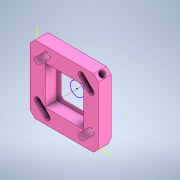
# Autodesk Inventor part: 20_Cube_Insert_Kinematic_Beautymirrormount_90_pro_v3
Saved by Autodesk Inventor 2022 (Build 260153000, 153)
## iProperties
Created: 2021-11-15
Part Number: 20_Cube_Insert_Kinematic_Beautymirrormount_90_pro_v3
Material: Generic
Document SubType Name: Modeling
Designer: diederichbenedict
Density: 1 g/cm^3
Appearance: Pink
Author: diederichbenedict
Autodesk Inventor part; units mm, degrees
ref_plane "YZ Plane" through (0, 0, 0) normal (1, 0, 0) x (0, 1, 0)
ref_plane "XY Plane" through (0, 0, 0) normal (0, 0, 1) x (1, 0, 0)
ref_plane "Work Plane1" through (0, 0, 2) normal (0, 0, 1) x (1, 0, 0)
sketch "Sketch1" plane through (0, 0, 2) normal (0, 0, 1) x (1, 0, 0)
  circle A0 centre (-37.0712, 14) radius 3.25 construction
  circle A1 centre (-9.0712, -14) radius 3.25 construction
  line L0 (-26.0712, -17.08) -> (-20.0712, -17.08) construction
  arc A2 (-20.0712, -17.08) -> (-20.0712, -14.08) centre (-20.0712, -15.58) ccw construction
  line L1 (-20.0712, -14.08) -> (-26.0712, -14.08) construction
  line L2 (-37.0712, -3) -> (-37.0712, 3) construction
  arc A3 (-37.0712, 3) -> (-40.0712, 3) centre (-38.5712, 3) ccw construction
  line L3 (-40.0712, 3) -> (-40.0712, -3) construction
  line L4 (-47.9712, -17) -> (-47.9712, 17) construction
  line L5 (-47.9712, 17) -> (-44.3964, 17) construction
  line L6 (-44.3964, 17) -> (-40.0712, 21.3252) construction
  line L7 (-40.0712, 21.3252) -> (-40.0712, 24.9) construction
  line L8 (-40.0712, 24.9) -> (-6.0712, 24.9) construction
  line L9 (-6.0712, 24.9) -> (-6.0712, 21.3252) construction
  line L10 (-6.0712, 21.3252) -> (-1.746, 17) construction
  line L11 (-1.746, 17) -> (1.8288, 17) construction
  line L12 (1.8288, 17) -> (1.8288, -17) construction
  line L13 (1.8288, -17) -> (-1.746, -17) construction
  line L14 (-1.746, -17) -> (-6.1126, -21.3666) construction
  line L15 (-6.1126, -21.3666) -> (-6.1126, -24.9) construction
  line L16 (-6.1126, -24.9) -> (-40.0712, -24.9) construction
  circle A4 centre (-37.0712, -14) radius 3.25 construction
  circle A5 centre (-23.0712, 0) radius 12.45 construction
  circle A6 centre (-23.0712, 0) radius 12.7 construction
  line L17 (-37.0712, 14) -> (-9.0712, 14) construction
  line L18 (-9.0712, 14) -> (-9.0712, -14) construction
  line L19 (-9.0712, -14) -> (-37.0712, -14) construction
  line L20 (-37.0712, -14) -> (-37.0712, 14) construction
  line L21 (-4.0712, -19) -> (-4.0712, 19)
  line L22 (-4.0712, 19) -> (-42.0712, 19)
  line L23 (-42.0712, 19) -> (-42.0712, -19)
  line L24 (-42.0712, -19) -> (-4.0712, -19)
  circle A7 centre (-23.0712, 0) radius 12.8
  circle A8 centre (-23.0712, 0) radius 3.25 projected
  line L25 (-40.0712, -24.9) -> (-40.0712, -21.3252) projected
  line L26 (-40.0712, -21.3252) -> (-44.3964, -17) projected
  line L27 (-44.3964, -17) -> (-47.9712, -17) projected
  arc A9 (-26.0712, -14.08) -> (-26.0712, -17.08) centre (-26.0712, -15.58) ccw projected
  arc A10 (-40.0712, -3) -> (-37.0712, -3) centre (-38.5712, -3) ccw projected
  circle A11 centre (-37.0712, -14) radius 3.25 projected
  point P0 (0, 0)
  point P1 (-21.8762, -3.0223)
  point P2 (-25.9925, 1.4242)
  dimension "d0" = 5
  dimension "d1" = 0.1
  constraints: 16 end point, 4 parallel, 2 perpendicular, 1 centre point, 1 horizontal, 3 other
  measures "d0" distance between parallel lines of L18 L21
  measures "d1" radial gap between concentric circles of A6 A7
extrude "Extrusion1" add sketch "Sketch1" along normal blind 6 contours L24 L23 L22 L21 | A7 | A11
sketch "Sketch2" plane through (0, 0, 2) normal (0, 0, -1) x (-1, 0, 0)
  circle A0 centre (23.0712, 0) radius 12.8 projected
  circle A1 centre (23.0712, 0) radius 8.5824
  point P0 (0, 0)
  constraints: 1 centre point
extrude "Extrusion2" add sketch "Sketch2" against normal blind 0.5
sketch "Sketch3" plane through (0, 0, 2) normal (0, 0, -1) x (-1, 0, 0)
  circle A0 centre (9.0712, -14) radius 1.45 construction
  circle A1 centre (9.0712, -14) radius 2.45
  circle A2 centre (37.0712, -14) radius 1.45 projected
  circle A3 centre (37.0712, -14) radius 1.95
  point P0 (0, 0)
  dimension "d8" = 1
  dimension "d10" = 0.5
  constraints: 2 centre point
  measures "d8" radial gap between concentric circles of A0 A1
  measures "d10" radial gap between concentric circles of A2 A3
sketch "Sketch5" plane through (0, 0, 2) normal (0, 0, -1) x (-1, 0, 0)
  arc A0 (20.0712, -14.08) -> (20.0712, -17.08) centre (20.0712, -15.58) ccw construction
  arc A1 (26.0712, -17.08) -> (26.0712, -14.08) centre (26.0712, -15.58) ccw construction
  line L0 (37.0712, 3) -> (37.0712, -3) projected
  arc A2 (37.0712, -3) -> (40.0712, -3) centre (38.5712, -3) ccw projected
  line L1 (40.0712, -3) -> (40.0712, 3) projected
  arc A3 (40.0712, 3) -> (37.0712, 3) centre (38.5712, 3) ccw projected
  line L2 (26.0712, -14.08) -> (20.0712, -14.08) construction
  arc A4 (20.0712, -14.08) -> (20.0712, -17.08) centre (20.0712, -15.58) ccw construction
  line L3 (20.0712, -17.08) -> (26.0712, -17.08) construction
  arc A5 (26.0712, -17.08) -> (26.0712, -14.08) centre (26.0712, -15.58) ccw construction
  circle A6 centre (37.0712, -14) radius 1.45 projected
  circle A7 centre (23.0712, 0) radius 1.45 projected
  circle A8 centre (9.0712, -14) radius 1.45 projected
  circle A9 centre (37.0712, 14) radius 1.45 projected
  line L4 (-1.8288, -17) -> (-1.8288, 17) projected
  line L5 (-1.8288, 17) -> (1.746, 17) projected
  line L6 (1.746, 17) -> (6.0712, 21.3252) projected
  line L7 (6.0712, 21.3252) -> (6.0712, 24.9) projected
  line L8 (6.0712, 24.9) -> (40.0712, 24.9) projected
  line L9 (40.0712, 24.9) -> (40.0712, 21.3252) projected
  line L10 (40.0712, 21.3252) -> (44.3964, 17) projected
  line L11 (44.3964, 17) -> (47.9712, 17) projected
  line L12 (47.9712, 17) -> (47.9712, -17) projected
  line L13 (44.3964, -17) -> (47.9712, -17) projected
  line L14 (40.0712, -21.3252) -> (44.3964, -17) projected
  line L15 (40.0712, -24.9) -> (40.0712, -21.3252) projected
  line L16 (6.1126, -24.9) -> (40.0712, -24.9) projected
  line L17 (6.1126, -24.9) -> (6.1126, -21.3666) projected
  line L18 (6.1126, -21.3666) -> (1.746, -17) projected
  line L19 (1.746, -17) -> (-1.8288, -17) projected
  line L20 (42.0712, -19) -> (4.0712, -19) projected
  arc A10 (9.5115, 9.1808) -> (9.5115, 7.0595) centre (10.5722, 8.1201) ccw
  arc A11 (16.0116, 11.4383) -> (16.0116, 13.5597) centre (14.951, 12.4989) ccw
  line L21 (16.0116, 11.4383) -> (11.6328, 7.0595)
  line L22 (14.8829, 12.4309) -> (10.6402, 8.1883) construction
  line L23 (9.5115, 9.1808) -> (13.8903, 13.5596)
  arc A12 (16.0116, 13.5597) -> (13.8903, 13.5596) centre (14.951, 12.4989) ccw
  arc A13 (9.5115, 7.0595) -> (11.6328, 7.0595) centre (10.5722, 8.1201) ccw
  arc A14 (16.0116, -13.5597) -> (16.0117, -11.4383) centre (14.951, -12.499) ccw
  arc A15 (13.8904, -13.5596) -> (16.0116, -13.5597) centre (14.951, -12.499) ccw
  line L24 (11.6329, -7.0595) -> (16.0117, -11.4383)
  line L25 (10.6402, -8.1883) -> (14.8829, -12.4309) construction
  arc A16 (11.6329, -7.0595) -> (9.5115, -7.0596) centre (10.5722, -8.1202) ccw
  line L26 (13.8904, -13.5596) -> (9.5116, -9.1808)
  arc A17 (9.5115, -7.0596) -> (9.5116, -9.1808) centre (10.5722, -8.1202) ccw
  arc A18 (36.6309, -7.0595) -> (34.5095, -7.0595) centre (35.5702, -8.1201) ccw
  arc A19 (36.6308, -9.1808) -> (36.6309, -7.0595) centre (35.5702, -8.1201) ccw
  line L27 (30.1307, -11.4383) -> (34.5095, -7.0595)
  line L28 (31.2595, -12.4309) -> (35.5021, -8.1883) construction
  arc A20 (30.1307, -11.4383) -> (30.1308, -13.5597) centre (31.1914, -12.4989) ccw
  line L29 (36.6308, -9.1808) -> (32.252, -13.5596)
  arc A21 (30.1308, -13.5597) -> (32.252, -13.5596) centre (31.1914, -12.4989) ccw
  arc A22 (30.1307, 13.5597) -> (30.1306, 11.4383) centre (31.1913, 12.499) ccw
  arc A23 (32.252, 13.5596) -> (30.1307, 13.5597) centre (31.1913, 12.499) ccw
  line L30 (34.5094, 7.0595) -> (30.1306, 11.4383)
  line L31 (35.5021, 8.1883) -> (31.2595, 12.4309) construction
  arc A24 (34.5094, 7.0595) -> (36.6308, 7.0596) centre (35.5701, 8.1202) ccw
  line L32 (32.252, 13.5596) -> (36.6308, 9.1808)
  arc A25 (36.6308, 7.0596) -> (36.6308, 9.1808) centre (35.5701, 8.1202) ccw
  point P0 (0, 0)
  point P1 (40.0712, -3)
  point P2 (9.9331, 8.8954)
  point P3 (14.1758, 13.138)
  point P4 (8.8725, 7.8347)
  point P5 (9.9331, 8.8954)
  point P6 (9.9331, 8.8954)
  point P7 (14.1758, 13.138)
  point P8 (15.2364, 14.1987)
  point P9 (18.0238, 11.4114)
  point P10 (14.1758, 13.138)
  point P11 (12.0544, 11.0167)
  point P12 (13.1151, 9.9561)
  point P13 (15.9025, 7.1687)
  point P14 (13.7811, 9.29)
  point P15 (11.7009, 11.3702)
  point P16 (15.9025, -7.1687)
  point P17 (15.2364, -14.1987)
  point P18 (14.1758, -13.138)
  point P19 (14.1758, -13.138)
  point P20 (14.1758, -13.138)
  point P21 (13.7811, -9.29)
  point P22 (13.1151, -9.9561)
  point P23 (11.701, -11.3702)
  point P24 (12.0544, -11.0167)
  point P25 (11.6598, -5.0474)
  point P26 (9.9331, -8.8954)
  point P27 (9.9331, -8.8954)
  point P28 (9.9331, -8.8954)
  point P29 (8.8725, -7.8347)
  point P30 (30.2399, -7.1687)
  point P31 (37.2699, -7.8347)
  point P32 (36.2092, -8.8954)
  point P33 (36.2092, -8.8954)
  point P34 (36.2092, -8.8954)
  point P35 (32.3612, -9.29)
  point P36 (33.0272, -9.9561)
  point P37 (34.4414, -11.3702)
  point P38 (34.0879, -11.0167)
  point P39 (28.1186, -11.4114)
  point P40 (31.9666, -13.138)
  point P41 (31.9666, -13.138)
  point P42 (31.9666, -13.138)
  point P43 (30.9059, -14.1987)
  point P44 (30.2399, 7.1687)
  point P45 (30.9059, 14.1987)
  point P46 (31.9666, 13.138)
  point P47 (31.9666, 13.138)
  point P48 (31.9666, 13.138)
  point P49 (32.3612, 9.29)
  point P50 (33.0272, 9.9561)
  point P51 (34.4414, 11.3702)
  point P52 (34.0879, 11.0167)
  point P53 (34.4825, 5.0474)
  point P54 (36.2092, 8.8954)
  point P55 (36.2092, 8.8954)
  point P56 (36.2092, 8.8954)
  point P57 (37.2699, 7.8347)
  point P58 (34.4414, -11.3702)
  point P59 (11.701, -11.3702)
  point P60 (34.4414, 11.3702)
  dimension "d133" = 360
  dimension "d139" = 1.5
  dimension "d140" = 1.5
  dimension "d141" = 3
  dimension "d144" = 360
  dimension "d146" = 32.1598
  dimension "d147" = 32.1598
  constraints: 32 point on circle, 16 centre point, 16 end point, 8 point on line, 143 other
  measures "d139" radius of A11
  measures "d140" radius of A10
  measures "d146" distance of point (34.441, -11.37) point (11.701, 11.37)
  measures "d147" distance of point (11.701, -11.37) point (34.441, 11.37)
extrude "Extrusion5" cut sketch "Sketch5" against normal blind 8 contours L23 A12 A11 L21 A13 A10 | A15 L26 A17 A16 L24 A14 | A19 L29 A21 A20 L27 A18 | A23 L32 A25 A24 L30 A22
sketch "Sketch6" plane through (-42.0712, -19, 8) normal (0, -1, 0) x (1, 0, 0)
  line L0 (0, -6) -> (38, -6) projected
  line L1 (38, -6) -> (38, 0) projected
  line L2 (0, 0) -> (38, 0) projected
  line L3 (0, -6) -> (0, 0) projected
  line L4 (31.8, 0) -> (31.8, 0) projected
  circle A0 centre (19, -3.5) radius 1.45
  point P0 (42.0712, -8)
  point P1 (4.5, 0)
  dimension "d34" = 2.9
  dimension "d126" = 2.5
  constraints: 1 centre point
  measures "d34" diameter of A0
  measures "d126" distance from line of L0 A0.centre
extrude "Extrusion6" [suppressed]
pattern_circular "Circular Pattern1" count 4 over 360 about axis through (-23.0712, 0, 2) along (0, 0, -1) of "Extrusion5"
chamfer "Chamfer1" distance 3 angle 45 4 edges at (-42.0712, 19, 5) (-4.0712, 19, 5) (-4.0712, -19, 5) (-42.0712, -19, 5)
sketch "Sketch13" plane through (0, 0, 2) normal (0, 0, -1) x (-1, 0, 0)
  circle A0 centre (23.0712, 0) radius 10.0484
  line L0 (42.0712, 16) -> (42.0712, -16) projected
  line L1 (39.0712, -19) -> (7.0712, -19) projected
  circle A1 centre (23.0712, 0) radius 3.25
  point P0 (0, 0)
  point P1 (42.0712, 0)
  point P2 (23.0712, -19)
  constraints: 2 centre point, 2 midpoint, 1 coincident, 1 horizontal alignment, 1 vertical alignment
hole "Hole1" at (-37.0712, -14, 2) direction (0, 0, 1) diameter 4 depth 0.1 tip angle 115
sketch "Sketch4" plane through (-4.0712, -19, 2) normal (1, 0, 0) x (0, 0, -1)
  line L0 (2, 4.45) -> (6, 4.45)
  line L1 (2, 1.55) -> (6, 1.55)
  line L2 (0, 0) -> (0, 38) projected
  arc A0 (2, 19) -> (2, 19) centre (1.5, 4.4206) ccw projected
  line L3 (-1.3741, 5) -> (-0.1, 7) projected
  line L4 (-1.3741, 5) -> (-0.1, 3) projected
  line L5 (-0.1, 7) -> (0.6045, 7)
  line L6 (0.6045, 7) -> (0.6045, 3)
  line L7 (0.6045, 3) -> (-0.1, 3)
  line L8 (-0.1, 3) -> (-0.1, 7)
  constraints: 12 end point, 3 horizontal, 2 parallel, 1 perpendicular, 4 other
extrude "Extrusion4" cut sketch "Sketch4" against normal blind 8 contours L7 L8 L5 L2 | L2 L5 L6 L7 | L4 L3 L8
sketch "Sketch9" plane through (-39.0712, 19, 2) normal (0, 1, 0) x (1, 0, 0)
  line L0 (35.8594, -6) -> (35.8594, -4)
  line L1 (35.8594, -4) -> (-5.4569, -4)
  line L2 (-5.4569, -4) -> (-5.4569, -6)
  line L3 (-5.4569, -6) -> (35.8594, -6)
  line L4 (32, -6) -> (0, -6) projected
  point P0 (39.0712, 2)
  dimension "d51" = 2
  constraints: 8 end point, 2 parallel, 1 collinear, 1 perpendicular, 1 vertical
  measures "d51" distance between parallel lines of L1 L3
extrude "Extrusion9" [suppressed]
sketch "Sketch11" plane through (0, 0, 2) normal (0, 0, -1) x (-1, 0, 0)
  circle A0 centre (23.0712, 0) radius 3.25 projected
  line L0 (12.0712, -16) -> (4.0712, -16) projected
  line L1 (7.0712, -19) -> (4.0712, -16) projected
  line L2 (39.0712, -19) -> (7.0712, -19) projected
  line L3 (42.0712, -16) -> (39.0712, -19) projected
  line L4 (42.0712, 16) -> (42.0712, -16) projected
  line L5 (39.0712, 19) -> (42.0712, 16) projected
  line L6 (7.0712, 19) -> (39.0712, 19) projected
  line L7 (4.0712, 16) -> (7.0712, 19) projected
  line L8 (4.0712, -12) -> (4.0712, 16) projected
  line L9 (4.0712, -12) -> (12.0712, -12) projected
  line L10 (12.0712, -12) -> (12.0712, -16) projected
  circle A1 centre (37.0712, -14) radius 2 projected
  circle A2 centre (23.0712, 0) radius 3.25 projected
  line L11 (4.0712, -12) -> (4.0712, 16) projected
  circle A3 centre (13.1721, 17.5) radius 1
  circle A4 centre (33.6721, 11) radius 1
  circle A5 centre (18.1721, -10.5) radius 1
  circle A6 centre (33.6721, 11) radius 0.9
  circle A7 centre (13.1721, 17.5) radius 0.9
  circle A8 centre (18.1721, -10.5) radius 0.9
  circle A9 centre (23.0712, 0) radius 7.071
  point P0 (0, 0)
  point P1 (0, 0)
  dimension "d57" = 1.8
  dimension "d58" = 1.8
  dimension "d59" = 1.8
  constraints: 7 centre point, 3 coincident
  measures "d57" diameter of A6
  measures "d58" diameter of A7
  measures "d59" diameter of A8
extrude "Extrusion10" [suppressed]
sketch "Sketch12" plane through (0, 0, 8) normal (0, 0, 1) x (1, 0, 0)
  line L0 (-32.0962, 9.025) -> (-14.0462, 9.025)
  line L1 (-14.0462, 9.025) -> (-14.0462, -9.025)
  line L2 (-14.0462, -9.025) -> (-32.0962, -9.025)
  line L3 (-32.0962, -9.025) -> (-32.0962, 9.025)
  line L4 (-7.0712, 19) -> (-39.0712, 19) projected
  line L5 (-4.0712, -16) -> (-4.0712, 16) projected
  point P0 (0, 0)
  point P1 (-23.0712, 9.025)
  point P2 (-23.0712, 19)
  point P3 (-14.0462, 0)
  point P4 (-4.0712, 0)
  dimension "d62" = 18.05
  dimension "d63" = 18.05
  constraints: 8 end point, 4 midpoint, 2 parallel, 1 horizontal, 1 horizontal alignment, 1 perpendicular, 1 vertical alignment
  measures "d62" distance of L0.start L0.end
  measures "d63" distance of L0.end L1.end
extrude "Extrusion11" cut sketch "Sketch12" against normal through all
sketch "Sketch14" plane through (0, 0, 8) normal (0, 0, 1) x (1, 0, 0)
  line L0 (-14.0462, 9.025) -> (-14.0462, -9.025) projected
  line L1 (-14.0462, -9.025) -> (-32.0962, -9.025) projected
  line L2 (-32.0962, -9.025) -> (-32.0962, 9.025) projected
  line L3 (-32.0962, 9.025) -> (-14.0462, 9.025) projected
  line L4 (-39.0712, -19) -> (-42.0712, -16) projected
  line L5 (-39.0712, -19) -> (-7.0712, -19) projected
  line L6 (-4.0712, -16) -> (-7.0712, -19) projected
  line L7 (-4.0712, -16) -> (-4.0712, 16) projected
  line L8 (-7.0712, 19) -> (-4.0712, 16) projected
  line L9 (-7.0712, 19) -> (-39.0712, 19) projected
  line L10 (-42.0712, 16) -> (-39.0712, 19) projected
  line L11 (-42.0712, 16) -> (-42.0712, -16) projected
  line L12 (-11.6328, 7.0595) -> (-16.0116, 11.4383) projected
  arc A0 (-13.8903, 13.5596) -> (-16.0116, 11.4383) centre (-14.951, 12.4989) ccw projected
  line L13 (-13.8903, 13.5596) -> (-9.5115, 9.1808) projected
  arc A1 (-11.6328, 7.0595) -> (-9.5115, 9.1808) centre (-10.5722, 8.1201) ccw projected
  line L14 (-16.0117, -11.4383) -> (-11.6329, -7.0595) projected
  arc A2 (-9.5116, -9.1808) -> (-11.6329, -7.0595) centre (-10.5722, -8.1202) ccw projected
  line L15 (-9.5116, -9.1808) -> (-13.8904, -13.5596) projected
  arc A3 (-16.0117, -11.4383) -> (-13.8904, -13.5596) centre (-14.951, -12.499) ccw projected
  line L16 (-34.5095, -7.0595) -> (-30.1307, -11.4383) projected
  arc A4 (-32.252, -13.5596) -> (-30.1307, -11.4383) centre (-31.1914, -12.4989) ccw projected
  line L17 (-32.252, -13.5596) -> (-36.6308, -9.1808) projected
  arc A5 (-34.5095, -7.0595) -> (-36.6308, -9.1808) centre (-35.5702, -8.1201) ccw projected
  line L18 (-30.1306, 11.4383) -> (-34.5094, 7.0595) projected
  arc A6 (-36.6308, 9.1808) -> (-34.5094, 7.0595) centre (-35.5701, 8.1202) ccw projected
  line L19 (-36.6308, 9.1808) -> (-32.252, 13.5596) projected
  arc A7 (-30.1306, 11.4383) -> (-32.252, 13.5596) centre (-31.1913, 12.499) ccw projected
  line L20 (-36.8212, 16) -> (-9.3212, 16)
  line L21 (-9.3212, 16) -> (-7.0712, 13.75)
  line L22 (-7.0712, 13.75) -> (-7.0712, -13.75)
  line L23 (-7.0712, -13.75) -> (-9.3212, -16)
  line L24 (-9.3212, -16) -> (-36.8212, -16)
  line L25 (-36.8212, -16) -> (-39.0712, -13.75)
  line L26 (-39.0712, -13.75) -> (-39.0712, 13.75)
  line L27 (-39.0712, 13.75) -> (-36.8212, 16)
  line L28 (-7.0712, 19) -> (-39.0712, 19) projected
  line L29 (-7.0712, 19) -> (-4.0712, 16) projected
  line L30 (-4.0712, -16) -> (-7.0712, -19) projected
  line L31 (-4.0712, -16) -> (-4.0712, 16) projected
  line L32 (-39.0712, -19) -> (-7.0712, -19) projected
  line L33 (-39.0712, -19) -> (-42.0712, -16) projected
  line L34 (-42.0712, 16) -> (-42.0712, -16) projected
  line L35 (-42.0712, 16) -> (-39.0712, 19) projected
  point P0 (-23.0712, 16)
  point P1 (-23.0712, 19)
  point P2 (-23.0712, -16)
  point P3 (-7.0712, 0)
  point P4 (-4.0712, 0)
  point P5 (-39.0712, 0)
  point P6 (-42.0712, 0)
  point P7 (-8.1962, -14.875)
  point P8 (-37.9462, 14.875)
  point P9 (-37.9462, -14.875)
  point P10 (-8.1962, 14.875)
  dimension "d190" = 27.5
  dimension "d194" = 3
  dimension "d195" = 3
  dimension "d196" = 3
  dimension "d197" = 3
  dimension "d198" = 27.5
  dimension "d199" = 27.5
  dimension "d200" = 27.5
  dimension "d201" = 3.182
  dimension "d202" = 3.182
  dimension "d203" = 3.182
  dimension "d204" = 3.182
  constraints: 16 end point, 11 midpoint, 10 parallel, 3 perpendicular, 2 horizontal alignment, 2 vertical alignment, 1 horizontal
  measures "d190" distance of L20.start L20.end
  measures "d194" distance between parallel lines of L20 L9
  measures "d195" distance between parallel lines of L7 L22
  measures "d196" distance between parallel lines of L5 L24
  measures "d197" distance between parallel lines of L11 L26
  measures "d198" distance of L21.end L22.end
  measures "d199" distance of L25.end L26.end
  measures "d200" distance of L23.end L24.end
  measures "d201" distance of L26.end L20.start
  measures "d202" distance of L20.end L21.end
  measures "d203" distance of L22.end L23.end
  measures "d204" distance of L24.end L25.end
extrude "Extrusion12" cut sketch "Sketch14" against normal blind 10 contours L20 L21 L22 L23 L24 L25 L26 L27 keep common part
sketch "Sketch16" plane through (0, 0, 2) normal (0, 0, -1) x (-1, 0, 0)
  line L0 (32.0962, 9.025) -> (14.0462, 9.025) projected
  line L1 (32.0962, 9.025) -> (14.0462, 9.025)
  line L2 (14.0462, 9.025) -> (14.0462, -9.025)
  line L3 (14.0462, -9.025) -> (32.0962, -9.025)
  line L4 (32.0962, -9.025) -> (32.0962, 9.025)
  line L5 (30.5962, 7.525) -> (15.5462, 7.525)
  line L6 (15.5462, 7.525) -> (15.5462, -7.525)
  line L7 (15.5462, -7.525) -> (30.5962, -7.525)
  line L8 (30.5962, -7.525) -> (30.5962, 7.525)
  point P0 (0, 0)
  point P1 (31.8369, 9.025)
  point P2 (14.3055, 9.025)
  point P3 (31.8369, 9.025)
  dimension "d120" = 1.5
  dimension "d121" = 1.5
  dimension "d122" = 1.5
  dimension "d123" = 1.5
  constraints: 16 end point, 4 parallel, 2 horizontal, 2 perpendicular
  measures "d120" distance between parallel lines of L8 L4
  measures "d121" distance between parallel lines of L7 L3
  measures "d122" distance between parallel lines of L2 L6
  measures "d123" distance between parallel lines of L0 L5
extrude "Extrusion14" add sketch "Sketch16" against normal blind 0.5
sketch "Sketch17" plane through (-36.4185, -16.4027, 8) normal (-0.7071068, -0.7071068, 0) x (-0.7071068, 0.7071068, 0)
  circle A0 centre (2.1213, 3) radius 1.45
  line L0 (4.2426, 6) -> (0, 6) projected
  point P0 (-14.1533, 8)
  point P1 (2.1213, 6)
  point P2 (2.1213, 6)
  dimension "d148" = 2.9
  dimension "d149" = 3
  constraints: 2 midpoint, 1 centre point, 1 vertical alignment
  measures "d148" diameter of A0
  measures "d149" distance of point (2.121, 6) A0.centre
extrude "Extrusion15" cut sketch "Sketch17" against normal blind 7
pattern_circular "Circular Pattern2" count 4 over 360 about axis through (-23.0712, 0, 2) along (0, 0, 1) of "Extrusion15"
equation "\"d63\" = d62"
body "Solid1"
